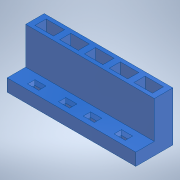
# Autodesk Inventor part: USB 3.0 A Recepticle Rear Insert Fit
Saved by Autodesk Inventor 2020.1 (Build 241239000, 239)
## iProperties
Created: 2019-11-21
Part Number: USB 3.0 A Recepticle Rear Insert Fit
Material: PBT Plastic
Document SubType Name: Modeling
Designer: S. Lee
Mass: 0.0740176 g
Surface Area: 2.4252 cm^2
Volume: 0.056502 cm^3
Density: 1.31 g/cm^3
Appearance: PBT Blue Pantone 300C
Author: S. Lee
Autodesk Inventor part; units mm, degrees
ref_plane "YZ Plane" through (0, 0, 0) normal (1, 0, 0) x (0, 1, 0)
ref_plane "XZ Plane" through (0, 0, 0) normal (0, 1, 0) x (-1, 0, 0)
ref_plane "XY Plane" through (0, 0, 0) normal (0, 0, 1) x (1, 0, 0)
sketch "Sketch1" plane through (0, 0, 0) normal (0, 1, 0) x (-1, 0, 0)
  line L0 (5.2, -1.5) -> (-5.2, -1.5)
  line L1 (-5.2, -1.5) -> (-5.2, 1.5)
  line L2 (-5.2, 1.5) -> (5.2, 1.5)
  line L3 (5.2, 1.5) -> (5.2, -1.5)
  line L4 (7.28, 0) -> (-7.28, 0) projected
  line L5 (0, -2.1) -> (0, 2.1) projected
  point P0 (0, 0)
  dimension "d0" = 10.4
  dimension "d1" = 3
  constraints: 8 end point, 2 parallel, 1 horizontal, 1 perpendicular, 2 other
  measures "d0" distance of L2.end L1.end
  measures "d1" distance of L1.end L0.end
extrude "Extrusion1" add sketch "Sketch1" along normal blind 4
sketch "Sketch2" plane through (0, 4, 0) normal (0, 1, 0) x (1, 0, 0)
  line L0 (-5.2, -1.5) -> (5.2, -1.5) projected
  line L1 (5.2, -1.5) -> (5.2, 1.5) projected
  line L2 (-5.2, -1.5) -> (5.2, -1.5)
  line L3 (5.2, -1.5) -> (5.2, 0)
  line L4 (5.2, 0) -> (-5.2, 0)
  line L5 (-5.2, 0) -> (-5.2, -1.5)
  line L6 (-4.75, 0.3) -> (-3.25, 0.3)
  line L7 (-3.25, 0.3) -> (-3.25, 1.2)
  line L8 (-3.25, 1.2) -> (-4.75, 1.2)
  line L9 (-4.75, 1.2) -> (-4.75, 0.3)
  line L10 (-5.2, 1.5) -> (-5.2, -1.5) projected
  line L11 (-2.75, 0.3) -> (-1.25, 0.3)
  line L12 (-1.25, 0.3) -> (-1.25, 1.2)
  line L13 (-1.25, 1.2) -> (-2.75, 1.2)
  line L14 (-2.75, 1.2) -> (-2.75, 0.3)
  line L15 (-0.75, 0.3) -> (0.75, 0.3)
  line L16 (0.75, 0.3) -> (0.75, 1.2)
  line L17 (0.75, 1.2) -> (-0.75, 1.2)
  line L18 (-0.75, 1.2) -> (-0.75, 0.3)
  line L19 (1.25, 0.3) -> (2.75, 0.3)
  line L20 (2.75, 0.3) -> (2.75, 1.2)
  line L21 (2.75, 1.2) -> (1.25, 1.2)
  line L22 (1.25, 1.2) -> (1.25, 0.3)
  line L23 (3.25, 0.3) -> (4.75, 0.3)
  line L24 (4.75, 0.3) -> (4.75, 1.2)
  line L25 (4.75, 1.2) -> (3.25, 1.2)
  line L26 (3.25, 1.2) -> (3.25, 0.3)
  point P0 (0, 0)
  dimension "d4" = 1.5
  dimension "d5" = 0.9
  dimension "d6" = 0.3
  dimension "d7" = 0.45
  dimension "d10" = 2
  constraints: 48 end point, 4 parallel, 3 horizontal, 2 perpendicular, 1 midpoint, 32 other
  measures "d4" distance of L8.end L7.end
  measures "d5" distance of L7.end L6.end
  measures "d6" distance between parallel lines of L4 L6
  measures "d7" distance between parallel lines of L10 L9
  measures "d10" distance of L6.start L11.start
extrude "Extrusion2" cut sketch "Sketch2" against normal blind 3
sketch "Sketch3" plane through (0, 1, 0) normal (0, 1, 0) x (1, 0, 0)
  line L0 (3.75, -0.9) -> (3.25, -0.9)
  line L1 (3.25, -0.9) -> (3.25, -0.7)
  line L2 (3.25, -0.7) -> (3.75, -0.7)
  line L3 (3.75, -0.7) -> (3.75, -0.9)
  line L4 (5.2, 1.5) -> (-5.2, 1.5) projected
  line L5 (5.2, -1.5) -> (-5.2, -1.5) projected
  line L6 (5.2, 0) -> (5.2, -1.5) projected
  line L7 (1.25, -0.9) -> (0.75, -0.9)
  line L8 (0.75, -0.9) -> (0.75, -0.7)
  line L9 (0.75, -0.7) -> (1.25, -0.7)
  line L10 (1.25, -0.7) -> (1.25, -0.9)
  line L11 (-0.75, -0.9) -> (-1.25, -0.9)
  line L12 (-1.25, -0.9) -> (-1.25, -0.7)
  line L13 (-1.25, -0.7) -> (-0.75, -0.7)
  line L14 (-0.75, -0.7) -> (-0.75, -0.9)
  line L15 (-3.25, -0.9) -> (-3.75, -0.9)
  line L16 (-3.75, -0.9) -> (-3.75, -0.7)
  line L17 (-3.75, -0.7) -> (-3.25, -0.7)
  line L18 (-3.25, -0.7) -> (-3.25, -0.9)
  line L19 (-5.2, -1.5) -> (-5.2, 0) projected
  line L20 (-3.75, 0.65) -> (-4.25, 0.65)
  line L21 (-4.25, 0.65) -> (-4.25, 0.85)
  line L22 (-4.25, 0.85) -> (-3.75, 0.85)
  line L23 (-3.75, 0.85) -> (-3.75, 0.65)
  line L24 (-4.75, 0.3) -> (-4.75, 1.2) projected
  line L25 (-3.25, 1.2) -> (-3.25, 0.3) projected
  line L26 (-4.75, 1.2) -> (-3.25, 1.2) projected
  line L27 (-3.25, 0.3) -> (-4.75, 0.3) projected
  line L28 (-1.75, 0.85) -> (-1.75, 0.65)
  line L29 (-1.75, 0.65) -> (-2.25, 0.65)
  line L30 (-2.25, 0.85) -> (-1.75, 0.85)
  line L31 (-2.25, 0.65) -> (-2.25, 0.85)
  line L32 (0.25, 0.85) -> (0.25, 0.65)
  line L33 (0.25, 0.65) -> (-0.25, 0.65)
  line L34 (-0.25, 0.85) -> (0.25, 0.85)
  line L35 (-0.25, 0.65) -> (-0.25, 0.85)
  line L36 (2.25, 0.85) -> (2.25, 0.65)
  line L37 (2.25, 0.65) -> (1.75, 0.65)
  line L38 (1.75, 0.85) -> (2.25, 0.85)
  line L39 (1.75, 0.65) -> (1.75, 0.85)
  line L40 (4.25, 0.85) -> (4.25, 0.65)
  line L41 (4.25, 0.65) -> (3.75, 0.65)
  line L42 (3.75, 0.85) -> (4.25, 0.85)
  line L43 (3.75, 0.65) -> (3.75, 0.85)
  point P0 (0, 0)
  dimension "d18" = 0.2
  dimension "d19" = 0.5
  dimension "d20" = 0.6
  dimension "d21" = 1.45
  dimension "d22" = 0.2
  dimension "d23" = 0.5
  dimension "d24" = 0.2
  dimension "d25" = 0.5
  dimension "d26" = 0.2
  dimension "d27" = 0.5
  dimension "d28" = 3.95
  dimension "d29" = 1.45
  dimension "d30" = 3.95
  dimension "d36" = 0.2
  dimension "d37" = 0.5
  dimension "d38" = 0.5
  dimension "d39" = 0.5
  dimension "d40" = 0.35
  dimension "d41" = 0.35
  dimension "d44" = 2
  constraints: 72 end point, 10 parallel, 6 horizontal, 5 perpendicular, 3 collinear, 32 other
  measures "d18" distance of L2.end L0.start
  measures "d19" distance of L1.end L2.end
  measures "d20" distance between parallel lines of L5 L0
  measures "d21" distance between parallel lines of L6 L3
  measures "d22" distance of L9.end L7.start
  measures "d23" distance of L8.end L9.end
  measures "d24" distance of L13.end L11.start
  measures "d25" distance of L12.end L13.end
  measures "d26" distance of L17.end L15.start
  measures "d27" distance of L16.end L17.end
  measures "d28" distance between parallel lines of L6 L10
  measures "d29" distance between parallel lines of L19 L16
  measures "d30" distance between parallel lines of L12 L19
  measures "d36" distance of L23.start L23.end
  measures "d37" distance of L22.start L23.start
  measures "d38" distance between parallel lines of L24 L21
  measures "d39" distance between parallel lines of L25 L23
  measures "d40" distance between parallel lines of L26 L22
  measures "d41" distance between parallel lines of L27 L20
  measures "d44" distance of L23.end L28.end
extrude "Extrusion3" cut sketch "Sketch3" against normal up to surface (1 mm away) contours L0 L1 L2 L3 | L7 L8 L9 L10 | L11 L12 L13 L14 | L15 L16 L17 L18 | L20 L21 L22 L23 | L28 L29 L31 L30 | L32 L33 L35 L34 | L36 L37 L39 L38 | L40 L41 L43 L42
chamfer "Chamfer1" distance 0.2 angle 45 36 edges at (-3.75, 1, 0.8) (-3.5, 1, 0.7) (-3.5, 1, 0.9) (-3.25, 1, 0.8) (-1.25, 1, 0.8) (-1, 1, 0.7) (-1, 1, 0.9) (-0.75, 1, 0.8) (0.75, 1, 0.8) (1, 1, 0.7) (1, 1, 0.9) (1.25, 1, 0.8) (3.25, 1, 0.8) (3.5, 1, 0.7) (3.5, 1, 0.9) (3.75, 1, 0.8) (3.75, 1, -0.75) (4, 1, -0.65) (4.25, 1, -0.75) (4, 1, -0.85) (2.25, 1, -0.75) (2, 1, -0.85) (1.75, 1, -0.75) (2, 1, -0.65) (0, 1, -0.65) (0.25, 1, -0.75) (-0.25, 1, -0.75) (0, 1, -0.85) (-1.75, 1, -0.75) (-2, 1, -0.85) (-2, 1, -0.65) (-2.25, 1, -0.75) (-3.75, 1, -0.75) (-4, 1, -0.85) (-4, 1, -0.65) (-4.25, 1, -0.75)
equation "\"d29\" = d21"
equation "\"d30\" = d28"
equation "\"d38\" = d39"
equation "\"d40\" = d41"
body "Solid1"
